Autodesk Fusion 360 part; units mm, degrees
note: some values were not read from the file. Chosen so that the rebuilt part matches the saved one: which bodies a step acts on; which face or edge a step refers to.
(part 2 of 2)
sketch "Sketch1" plane through (0, 0, 0) normal (0, 0, 1) x (1, 0, 0)
  circle A0 centre (0, 0) radius 6.5
  dimension "d1" = 13
  constraint coincident A0.centre origin
  measures "d1" diameter of A0
extrude "Extrude1" add sketch "Sketch1" along normal blind 5 makes body 1
sketch "Sketch2" plane through (0, 0, 5) normal (0, 0, 1) x (-1, 0, 0)
  circle A0 centre (0, 0) radius 6.5
  circle A1 centre (0, 0) radius 5.3449
  circle A2 centre (0, 0) radius 2
  circle A3 centre (0, 0) radius 3.2776
  circle A4 centre (0, 0) radius 3.3825
  circle A5 centre (0, 0) radius 5.248
  dimension "d4" = 4
  constraint concentric A0 A1
  constraint concentric A1 A2
  constraint concentric A1 A3
  constraint concentric A3 A4
  constraint concentric A2 A5
  measures "d4" diameter of A2
extrude "Extrude2" cut sketch "Sketch2" against normal blind 10 contours A2 bodies 1
extrude "Extrude3" cut sketch "Sketch2" against normal blind 0.3 contours A1 | A4 bodies 1
extrude "Extrude4" cut sketch "Sketch2" against normal blind 0.1 contours A3 | A5 bodies 1
extrude "Extrude5" cut 1 faces at (4.9684, -0.4223, 0) along direction (0, 0, 1) blind 2.5 on bodies 1 bodies 1
mirror "Mirror1" about plane through (0, 0, 2.5) normal (0, 0, -1) of bodies 1 makes body 2
combine "Combine1" operation add target body 2 tool bodies 1
copy_body "Body->Comp1" bodies 2 removing the originals makes body 3 in component "4mmBearing"
chamfer "Chamfer1" distance 0.25 angle 45 2 edges at (-6.0601, -2.3505, 5) (-6.0601, -2.3505, 0) on bodies 3 in component "4mmBearing"
chamfer "Chamfer2" distance 0.2 angle 45 2 edges at (1.8647, 0.7232, 0.1) (1.8647, 0.7232, 4.9) on bodies 3 in component "4mmBearing"
component "4mmBearing" placed x (1, 0, 0) y (0, 1, 0) z (0, 0, 1) at (0, 0, 0)
